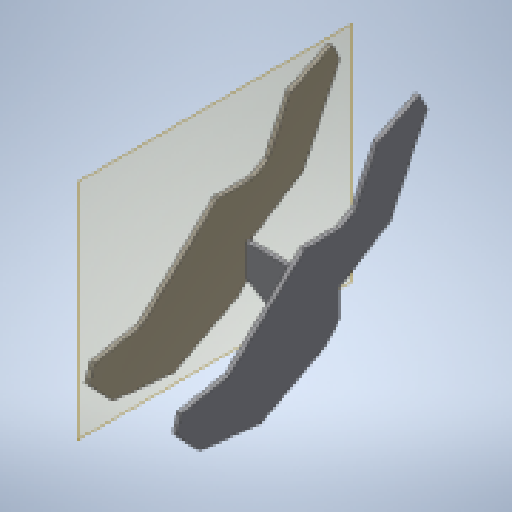
# Autodesk Inventor part: ShoulderCollision
Saved by Autodesk Inventor 2023 (Build 270158000, 158)
## iProperties
Created: 2023-03-28
Part Number: ShoulderCollision
Material: Generic
Document SubType Name: Modeling
Designer: LattePanda
Density: 1 g/cm^3
Appearance: Default
Author: LattePanda
Autodesk Inventor part; units mm, degrees
sketch "Sketch1" plane through (0, 0, 0) normal (0, 0, 1) x (1, 0, 0)
  circle A0 centre (0, 0) radius 10.16
  arc A1 (-9.6844, 3.0721) -> (-9.6844, -3.0721) centre (0, 0) ccw construction
  constraints: 1 centre point, 1 coincident, 1 concentric
ref_plane "Work Plane1" through (-24.1297, -20.1241, 6.985) normal (0, 0, -1) x (0, 1, 0)
extrude "Extrusion1" add sketch "Sketch1" along normal up to surface (6.985 mm away)
sketch "Sketch2" plane through (0, 0, 6.985) normal (0, 0, 1) x (1, 0, 0)
  line L0 (-24.1297, 19.05) -> (24.1297, 19.05) construction
  line L1 (-30.4797, 4.9571) -> (-30.4797, 51.5313) construction
  line L2 (30.4797, 51.5313) -> (30.4797, 4.9571) construction
  line L3 (-3.5464, -20.1241) -> (3.5464, -20.1241)
  line L4 (3.5464, -20.1241) -> (30.4797, -3.81)
  line L5 (-3.5464, -20.1241) -> (-30.4797, -3.81)
  line L6 (-30.4797, -3.81) -> (-30.4797, 19.05)
  line L7 (-30.4797, 19.05) -> (30.4797, 19.05)
  line L8 (30.4797, 19.05) -> (30.4797, -3.81)
  line L9 (0, 141.501) -> (0, -68.047)
  arc A0 (-6.5797, -18.2867) -> (6.5797, -18.2867) centre (0, -7.4241) ccw construction
  line L10 (-6.5797, -18.2867) -> (-24.1297, -7.6563) construction
  line L11 (24.1297, -7.6563) -> (6.5797, -18.2867) construction
  point P0 (0, 0)
  point P1 (0, -20.1241)
  constraints: 14 end point, 5 collinear, 2 perpendicular, 2 vertical, 1 horizontal, 1 midpoint, 1 point on line, 1 tangent, 2 other
ref_plane "Work Plane2" through (-24.1297, -20.1241, 10.16) normal (0, 0, 1) x (1, 0, 0)
extrude "Extrusion2" add sketch "Sketch2" along normal up to surface (3.175 mm away)
ref_plane "Work Plane3" through (-30.4797, 28.613, 25.8435) normal (1, 0, 0) x (0, 1, -0.0012)
sketch "Sketch3" plane through (-30.4797, 28.613, 25.8435) normal (1, 0, 0) x (0, 1, -0.0012)
  line L0 (-60.3032, 83.7671) -> (-46.2664, 96.8991) construction
  line L1 (-40.061, 98.3138) -> (-35.1427, 96.7719) construction
  line L2 (-30.8232, 91.9054) -> (-25.3621, 62.7037) construction
  line L3 (-66.4956, 38.9741) -> (-62.271, 79.8043) construction
  line L4 (-41.8663, -9.4545) -> (-65.7822, 35.3495) construction
  line L5 (-23.7279, 59.5092) -> (22.9055, 10.5268) construction
  line L6 (28.1348, -2.5269) -> (28.1554, -19.5123) construction
  line L7 (-12.3805, -21.1807) -> (-26.3576, -21.2033) construction
  line L8 (-30.4769, -19.6947) -> (-40.5808, -11.1193) construction
  line L9 (13.7735, -56.6336) -> (-7.0203, -24.1102) construction
  line L10 (69.8762, -83.775) -> (16.4352, -58.9603) construction
  line L11 (28.9647, -22.6068) -> (33.5205, -30.7438) construction
  line L12 (36.3869, -33.401) -> (67.1857, -47.7021) construction
  line L13 (70.2201, -50.6979) -> (81.3231, -73.8278) construction
  line L14 (78.362, -82.2562) -> (75.2702, -83.7404) construction
  line L15 (-62.0279, 82.1535) -> (-43.5762, 99.4159)
  line L16 (-43.5762, 99.4159) -> (-31.521, 95.6364)
  line L17 (-31.521, 95.6364) -> (-25.0181, 60.8644)
  line L18 (-25.0181, 60.8644) -> (28.1257, 5.0437)
  line L19 (28.1257, 5.0437) -> (28.1574, -21.1648)
  line L20 (28.1574, -21.1648) -> (34.5239, -32.536)
  line L21 (34.5239, -32.536) -> (69.2399, -48.656)
  line L22 (69.2399, -48.656) -> (84.0568, -79.5226)
  line L23 (84.0568, -79.5226) -> (72.5814, -85.0311)
  line L24 (72.5814, -85.0311) -> (14.7653, -58.1848)
  line L25 (14.7653, -58.1848) -> (-8.8968, -21.1751)
  line L26 (-8.8968, -21.1751) -> (-28.6949, -21.2071)
  line L27 (-28.6949, -21.2071) -> (-41.3065, -10.5034)
  line L28 (-41.3065, -10.5034) -> (-66.6939, 37.0577)
  line L29 (-66.6939, 37.0577) -> (-62.0279, 82.1535)
  point P0 (-28.5817, -25.8781)
  constraints: 30 end point, 15 collinear, 1 parallel
ref_plane "Work Plane4" through (-33.6547, -38.1116, -58.8269) normal (-1, 0, 0) x (0, 0.0012, 1)
extrude "Extrusion3" add sketch "Sketch3" against normal up to surface (3.175 mm away)
mirror "Mirror1" about plane through (0, 0, 0) normal (1, 0, 0) of "Extrusion3"
body "Solid1"
